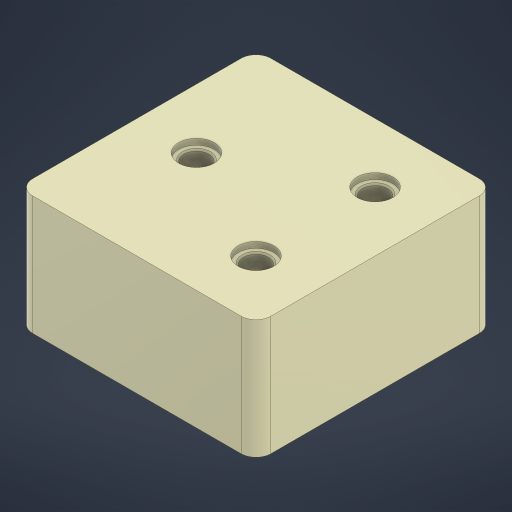
# Autodesk Inventor part: Tool_Holder
Saved by Autodesk Inventor 2023 (Build 270158000, 158)
## iProperties
Created: 2023-03-09
Part Number: Tool_Holder
Material: ABS Plastic
Document SubType Name: Modeling
Designer: dzw04
Density: 1.06 g/cm^3
Appearance: Smooth - Ash
Author: dzw04
Autodesk Inventor part; units mm, degrees
ref_plane "YZ Plane" through (0, 0, 0) normal (1, 0, 0) x (0, 1, 0)
ref_plane "XZ Plane" through (0, 0, 0) normal (0, 1, 0) x (-1, 0, 0)
ref_plane "XY Plane" through (0, 0, 0) normal (0, 0, 1) x (1, 0, 0)
sketch "Sketch1" plane through (0, 0, 0) normal (0, 1, 0) x (-1, 0, 0)
  line L0 (-20, 20) -> (20, 20)
  line L1 (20, 20) -> (20, -20)
  line L2 (20, -20) -> (-20, -20)
  line L3 (-20, -20) -> (-20, 20)
  line L4 (-20, 20) -> (20, -20) construction
  line L5 (20, 20) -> (-20, -20) construction
  line L6 (20, 0) -> (10, 0) construction
  circle A0 centre (10, 0) radius 2.1
  line L7 (10, 0) -> (0, 0) construction
  line L8 (0, 0) -> (-10, 0) construction
  line L9 (-10, 0) -> (-10, -10) construction
  line L10 (-10, -10) -> (-10, 10) construction
  circle A1 centre (-10, 10) radius 2.1
  circle A2 centre (-10, -10) radius 2.1
  dimension "d0" = 40
  dimension "d1" = 40
  dimension "d2" = 10
  dimension "d3" = 4.2
  dimension "d4" = 10
  dimension "d5" = 10
  dimension "d6" = 10
  dimension "d7" = 20
  dimension "d8" = 4.2
  dimension "d9" = 4.2
  constraints: 22 end point, 3 centre point, 3 coincident, 3 horizontal, 3 midpoint, 3 point on line, 2 parallel, 1 perpendicular
  measures "d0" distance of L1.end L2.end
  measures "d1" distance of L0.end L1.end
  measures "d2" distance of L6.start L6.end
  measures "d3" diameter of A0
  measures "d4" distance of L7.start L7.end
  measures "d5" distance of L7.end L8.end
  measures "d6" distance of L8.end L9.end
  measures "d7" distance of L9.end L10.end
  measures "d8" diameter of A1
  measures "d9" diameter of A2
extrude "Extrusion1" add sketch "Sketch1" along normal blind 20
sketch "Sketch2" plane through (0, 20, 0) normal (0, 1, 0) x (1, 0, 0)
  circle A0 centre (-10, 0) radius 2.1 projected
  circle A1 centre (-10, 0) radius 3
  circle A2 centre (10, 10) radius 2.1 projected
  circle A3 centre (10, 10) radius 3
  circle A4 centre (10, -10) radius 2.1 projected
  circle A5 centre (10, -10) radius 3
  point P0 (0, 0)
  dimension "d12" = 6
  dimension "d13" = 6
  dimension "d14" = 6
  constraints: 3 centre point, 3 coincident
  measures "d12" diameter of A1
  measures "d13" diameter of A3
  measures "d14" diameter of A5
extrude "Extrusion2" cut sketch "Sketch2" against normal blind 1 contours A0 | A1 | A2 | A3 | A4 | A5
sketch "Sketch3" plane through (0, 0, 0) normal (0, -1, 0) x (1, 0, 0)
  circle A0 centre (-10, 0) radius 2.1 projected
  circle A1 centre (-10, 0) radius 3
  circle A2 centre (10, 10) radius 3 projected
  circle A3 centre (10, 10) radius 3
  circle A4 centre (10, -10) radius 2.1 projected
  circle A5 centre (10, -10) radius 3
  point P0 (0, 0)
  dimension "d17" = 6
  dimension "d18" = 6
  dimension "d19" = 6
  constraints: 3 centre point, 3 coincident
  measures "d17" diameter of A1
  measures "d18" diameter of A3
  measures "d19" diameter of A5
extrude "Extrusion3" cut sketch "Sketch3" against normal blind 1 contours A0 | A1 | A2 | A4 | A5
chamfer "Chamfer1" distance 0.25 angle 45 6 edges at (12.1, 1, 10) (-7.9, 1, 0) (12.1, 1, -10) (12.1, 19, -10) (-7.9, 19, 0) (12.1, 19, 10)
sketch "Sketch4" plane through (-20, 0, -20) normal (-1, 0, 0) x (0, 0, 1)
  line L0 (40, 20) -> (0, 20) construction
  line L1 (20, 20) -> (20, 0) construction
  line L2 (20, 10) -> (27.5, 10) construction
  line L3 (27.5, 10) -> (12.5, 10) construction
  circle A0 centre (12.5, 10) radius 2.1
  circle A1 centre (27.5, 10) radius 2.1
  dimension "d25" = 7.5
  dimension "d26" = 15
  dimension "d27" = 4.2
  dimension "d28" = 4.2
  constraints: 6 end point, 2 centre point, 2 coincident, 2 midpoint, 1 horizontal, 1 point on line, 1 vertical
  measures "d25" distance of L2.start L2.end
  measures "d26" distance of L2.end L3.end
  measures "d27" diameter of A0
  measures "d28" diameter of A1
extrude "Extrusion4" cut sketch "Sketch4" against normal blind 15
sketch "Sketch5" plane through (-20, 0, -20) normal (-1, 0, 0) x (0, 0, 1)
  circle A0 centre (12.5, 10) radius 2.1 projected
  circle A1 centre (12.5, 10) radius 3
  circle A2 centre (27.5, 10) radius 2.1 projected
  circle A3 centre (27.5, 10) radius 3
  point P0 (20, 0)
  dimension "d31" = 6
  dimension "d32" = 6
  constraints: 2 centre point, 2 coincident
  measures "d31" diameter of A1
  measures "d32" diameter of A3
extrude "Extrusion5" cut sketch "Sketch5" against normal blind 1 contours A0 | A1 | A2 | A3
chamfer "Chamfer2" distance 0.25 angle 45 2 edges at (-19, 10, -9.6) (-19, 10, 5.4)
fillet "Fillet1" radius 2.5 4 edges at (-20, 10, -20) (-20, 10, 20) (20, 10, 20) (20, 10, -20)
sketch "Sketch6" plane through (-20, 0, -17.5) normal (-1, 0, 0) x (0, 0, 1)
  line L0 (14.5, 20) -> (20.5, 20) construction
  line L1 (17.5, 20) -> (17.5, 0) construction
  circle A0 centre (17.5, 10) radius 2.1
  line L2 (17.5, 10) -> (32.5, 10) construction
  line L3 (35, 20) -> (35, 0) projected
  circle A1 centre (32.5, 10) radius 2.1
  line L4 (17.5, 10) -> (2.5, 10) construction
  circle A2 centre (2.5, 10) radius 2.1
  dimension "d39" = 4.2
  dimension "d40" = 15
  dimension "d41" = 4.2
  dimension "d43" = 15
  dimension "d44" = 4.2
  constraints: 6 end point, 3 centre point, 2 coincident, 2 midpoint, 1 horizontal, 1 perpendicular, 1 vertical
  measures "d39" diameter of A0
  measures "d40" distance of L2.start L2.end
  measures "d41" diameter of A1
  measures "d43" distance of L2.start L4.end
  measures "d44" diameter of A2
extrude "Extrusion6" cut sketch "Sketch6" against normal up to surface (15 mm away)
sketch "Sketch7" plane through (-20, 0, -17.5) normal (-1, 0, 0) x (0, 0, 1)
  circle A0 centre (2.5, 10) radius 2.1 projected
  circle A1 centre (2.5, 10) radius 3
  circle A2 centre (17.5, 10) radius 2.1 projected
  circle A3 centre (17.5, 10) radius 3
  circle A4 centre (32.5, 10) radius 2.1 projected
  circle A5 centre (32.5, 10) radius 3
  point P0 (17.5, 0)
  dimension "d47" = 6
  dimension "d48" = 6
  dimension "d49" = 6
  constraints: 3 centre point, 3 coincident
  measures "d47" diameter of A1
  measures "d48" diameter of A3
  measures "d49" diameter of A5
extrude "Extrusion7" cut sketch "Sketch7" against normal blind 1 contours A0 | A1 | A3 | A4 | A5
body "Solid1"
